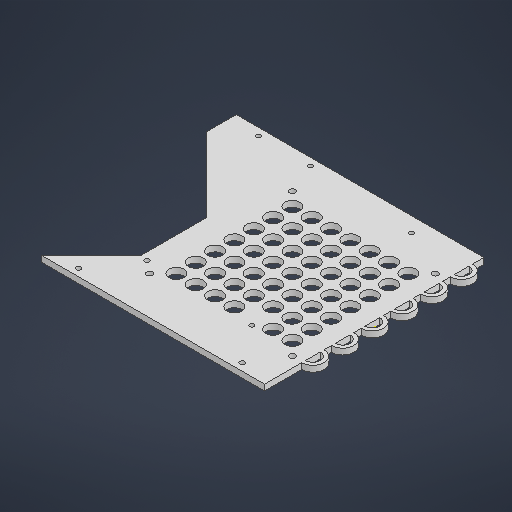
# Autodesk Inventor part: SidePlate_Ebox
Saved by Autodesk Inventor 2025.1 (Build 291241000, 241)
## iProperties
Created: 2025-03-19
Part Number: SidePlate_Ebox
Material: Generic
Document SubType Name: Modeling
Designer: m_kni
Density: 1 g/cm^3
Appearance: Default
Author: m_kni
Autodesk Inventor part; units mm, degrees
ref_plane "YZ Plane" through (0, 0, 0) normal (1, 0, 0) x (0, 1, 0)
ref_plane "XZ Plane" through (0, 0, 0) normal (0, 1, 0) x (-1, 0, 0)
ref_plane "XY Plane" through (0, 0, 0) normal (0, 0, 1) x (1, 0, 0)
sketch "Sketch1" plane through (0, 0, 0) normal (0, 1, 0) x (-1, 0, 0)
  line L0 (-83.0918, 73.8924) -> (-83.0918, -73.6076)
  line L1 (-83.0918, 73.8924) -> (-83.0918, -73.6076)
  line L2 (66.9082, 73.8924) -> (-83.0918, 73.8924)
  line L3 (-83.0918, 73.8924) -> (-83.0918, -73.6076)
  line L4 (-83.0918, -73.6076) -> (83.4082, -73.6076)
  line L5 (83.4082, -73.6076) -> (83.4082, -53.6076)
  line L6 (83.4082, -53.6076) -> (33.4082, -3.6076)
  line L7 (33.4082, -3.6076) -> (33.4082, 40.3924)
  line L8 (33.4082, 40.3924) -> (66.9082, 73.8924)
  point P0 (0, 0)
  point P1 (-8.0918, 73.8924)
  constraints: 18 end point, 1 vertical
extrude "Extrusion1" add sketch "Sketch1" along normal blind 4
sketch "Sketch2" plane through (0, 4, 0) normal (0, 1, 0) x (1, 0, 0)
  line L0 (83.0918, -73.8924) -> (83.0918, 73.6076) projected
  line L1 (-66.9082, -73.8924) -> (83.0918, -73.8924) projected
  line L2 (83.0918, -73.8924) -> (-66.9082, -73.8924)
  circle A0 centre (-46.9082, -68.8924) radius 1.6
  circle A1 centre (63.0918, -68.8924) radius 1.6
  point P0 (0, 0)
  dimension "d2" = 20
  dimension "d3" = 5
  dimension "d4" = 20
  dimension "d5" = 3.2
  dimension "d6" = 3.2
  constraints: 2 centre point, 2 coincident, 2 end point, 1 collinear
  measures "d2" horizontal distance of point (-46.908, -68.892) L1.start
  measures "d3" distance from line of L1 point (-46.908, -68.892)
  measures "d4" distance from line of point (63.092, -68.892) L0
  measures "d5" diameter of A0
  measures "d6" diameter of A1
extrude "Extrusion2" cut sketch "Sketch2" against normal blind 10
sketch "Sketch3" plane through (0, 4, 0) normal (0, 1, 0) x (1, 0, 0)
  line L0 (83.0918, 73.6076) -> (-83.4082, 73.6076) projected
  line L1 (-83.4082, 73.6076) -> (-83.4082, 53.6076) projected
  circle A0 centre (-63.4082, 68.6076) radius 1.5
  circle A1 centre (-28.4082, 68.6076) radius 1.5
  circle A2 centre (-28.4082, -41.3924) radius 1.5
  point P0 (0, 0)
  dimension "d9" = 5
  dimension "d10" = 20
  dimension "d11" = 3
  dimension "d12" = 35
  dimension "d13" = 110
  dimension "d14" = 3
  dimension "d15" = 3
  constraints: 3 centre point, 3 coincident
  measures "d9" distance from line of point (-63.408, 68.608) L0
  measures "d10" distance from line of L1 point (-63.408, 68.608)
  measures "d11" diameter of A0
  measures "d12" distance of point (-28.408, 68.608) A0.centre
  measures "d13" distance of point (-28.408, -41.392) point (-28.408, 68.608)
  measures "d14" diameter of A1
  measures "d15" diameter of A2
extrude "Extrusion3" cut sketch "Sketch3" against normal blind 10
sketch "Sketch4" plane through (0, 4, 0) normal (0, 1, 0) x (1, 0, 0)
  line L0 (83.0918, -73.8924) -> (83.0918, 73.6076) projected
  line L1 (-66.9082, -73.8924) -> (83.0918, -73.8924) projected
  circle A0 centre (44.5918, 63.6076) radius 1.5
  circle A1 centre (44.5918, -43.8924) radius 1.5
  point P0 (0, 0)
  dimension "d18" = 38.5
  dimension "d19" = 30
  dimension "d20" = 107.5
  dimension "d21" = 3
  dimension "d22" = 3
  constraints: 2 centre point, 2 coincident
  measures "d18" distance from line of L0 point (44.592, -43.892)
  measures "d19" distance from line of point (44.592, -43.892) L1
  measures "d20" distance of point (44.592, 63.608) point (44.592, -43.892)
  measures "d21" diameter of A0
  measures "d22" diameter of A1
extrude "Extrusion4" cut sketch "Sketch4" against normal blind 10
sketch "Sketch5" plane through (0, 4, 0) normal (0, 1, 0) x (1, 0, 0)
  line L0 (83.0918, -73.8924) -> (83.0918, 73.6076) projected
  line L1 (83.0918, -0.1424) -> (-26.9082, -0.1424)
  line L2 (-33.4082, 3.6076) -> (-33.4082, -40.3924) projected
  line L3 (83.0918, -55.1424) -> (-26.9082, -55.1424)
  line L4 (-26.9082, -55.1424) -> (-26.9082, 54.8576)
  line L5 (-26.9082, 54.8576) -> (83.0918, 54.8576)
  line L6 (83.0918, 54.8576) -> (83.0918, -55.1424)
  line L7 (83.0918, -55.1424) -> (-26.9082, 54.8576) construction
  line L8 (-26.9082, -55.1424) -> (83.0918, 54.8576) construction
  line L9 (76.0918, -48.1424) -> (-19.9082, -48.1424)
  line L10 (-19.9082, -48.1424) -> (-19.9082, 47.8576)
  line L11 (-19.9082, 47.8576) -> (76.0918, 47.8576)
  line L12 (76.0918, 47.8576) -> (76.0918, -48.1424)
  line L13 (76.0918, -48.1424) -> (-19.9082, 47.8576) construction
  line L14 (-19.9082, -48.1424) -> (76.0918, 47.8576) construction
  circle A0 centre (-19.9082, 47.8576) radius 2
  circle A1 centre (76.0918, 47.8576) radius 2
  circle A2 centre (-19.9082, -48.1424) radius 2
  circle A3 centre (76.0918, -48.1424) radius 2
  circle A4 centre (-11.0143, 38.9637) radius 5
  circle A5 centre (-11.0143, 25.9637) radius 5
  circle A6 centre (-11.0143, 12.9637) radius 5
  circle A7 centre (-11.0143, -0.0363) radius 5
  circle A8 centre (-11.0143, -13.0363) radius 5
  circle A9 centre (-11.0143, -26.0363) radius 5
  circle A10 centre (-11.0143, -39.0363) radius 5
  circle A11 centre (1.9857, 38.9637) radius 5
  circle A12 centre (1.9857, 25.9637) radius 5
  circle A13 centre (1.9857, 12.9637) radius 5
  circle A14 centre (1.9857, -0.0363) radius 5
  circle A15 centre (1.9857, -13.0363) radius 5
  circle A16 centre (1.9857, -26.0363) radius 5
  circle A17 centre (1.9857, -39.0363) radius 5
  circle A18 centre (14.9857, 38.9637) radius 5
  circle A19 centre (14.9857, 25.9637) radius 5
  circle A20 centre (14.9857, 12.9637) radius 5
  circle A21 centre (14.9857, -0.0363) radius 5
  circle A22 centre (14.9857, -13.0363) radius 5
  circle A23 centre (14.9857, -26.0363) radius 5
  circle A24 centre (14.9857, -39.0363) radius 5
  circle A25 centre (27.9857, 38.9637) radius 5
  circle A26 centre (27.9857, 25.9637) radius 5
  circle A27 centre (27.9857, 12.9637) radius 5
  circle A28 centre (27.9857, -0.0363) radius 5
  circle A29 centre (27.9857, -13.0363) radius 5
  circle A30 centre (27.9857, -26.0363) radius 5
  circle A31 centre (27.9857, -39.0363) radius 5
  circle A32 centre (40.9857, 38.9637) radius 5
  circle A33 centre (40.9857, 25.9637) radius 5
  circle A34 centre (40.9857, 12.9637) radius 5
  circle A35 centre (40.9857, -0.0363) radius 5
  circle A36 centre (40.9857, -13.0363) radius 5
  circle A37 centre (40.9857, -26.0363) radius 5
  circle A38 centre (40.9857, -39.0363) radius 5
  circle A39 centre (53.9857, 38.9637) radius 5
  circle A40 centre (53.9857, 25.9637) radius 5
  circle A41 centre (53.9857, 12.9637) radius 5
  circle A42 centre (53.9857, -0.0363) radius 5
  circle A43 centre (53.9857, -13.0363) radius 5
  circle A44 centre (53.9857, -26.0363) radius 5
  circle A45 centre (53.9857, -39.0363) radius 5
  circle A46 centre (66.9857, 38.9637) radius 5
  circle A47 centre (66.9857, 25.9637) radius 5
  circle A48 centre (66.9857, 12.9637) radius 5
  circle A49 centre (66.9857, -0.0363) radius 5
  circle A50 centre (66.9857, -13.0363) radius 5
  circle A51 centre (66.9857, -26.0363) radius 5
  circle A52 centre (66.9857, -39.0363) radius 5
  point P0 (0, 0)
  point P1 (28.0918, -0.1424)
  dimension "d25" = 110
  dimension "d26" = 110
  dimension "d27" = 96
  dimension "d28" = 96
  dimension "d29" = 4
  dimension "d30" = 4
  dimension "d31" = 4
  dimension "d32" = 4
  dimension "d33" = 10
  dimension "d36" = 13
  dimension "d39" = 13
  constraints: 53 centre point, 26 end point, 6 midpoint, 4 coincident, 4 parallel, 3 horizontal, 3 perpendicular, 1 point on line, 1 vertical, 96 other
  measures "d25" distance of L1.start L1.end
  measures "d26" distance of L3.end L4.end
  measures "d27" distance of L10.end L11.end
  measures "d28" distance of L9.end L10.end
  measures "d29" diameter of A0
  measures "d30" diameter of A1
  measures "d31" diameter of A2
  measures "d32" diameter of A3
  measures "d33" diameter of A4
  measures "d36" distance of A4.centre A5.centre
  measures "d39" distance of A4.centre A11.centre
extrude "Extrusion5" cut sketch "Sketch5" against normal blind 10 contours A49 L1 | L1 A49 | A1 L11 L12 | L12 L11 A1 | A3 L9 L12 | L12 L9 A3 | A7 L1 | L1 A7 | A2 L9 L10 | L10 L9 A2 | A0 L11 L10 | L10 L11 A0 | A42 L1 | L1 A42 | A14 L1 | L1 A14 | A35 L1 | L1 A35 | A21 L1 | L1 A21 | A28 L1 | L1 A28 | A4 | A5 | A6 | A8 | A9 | A10 | A11 | A12 | A13 | A15 | A16 | A17 | A18 | A19 | A20 | A22 | A23 | A24 | A25 | A26 | A27 | A29 | A30 | A31 | A32 | A33 | A34 | A36 | A37 | A39 | A40 | A41 | A43 | A44 | A45 | A46 | A47 | A48 | A50 | A51 | A52
sketch "Sketch6" plane through (83.0918, 0, 73.8924) normal (1, 0, 0) x (0, 0, -1)
  point P0 (73.8924, 0)
sketch "Sketch7" plane through (0, 4, 0) normal (0, 1, 0) x (1, 0, 0)
  line L0 (83.0918, -73.8924) -> (83.0918, 73.6076) projected
  line L1 (83.0918, 73.6076) -> (-83.4082, 73.6076) projected
  circle A0 centre (83.0918, 58.6076) radius 5
  circle A1 centre (83.0918, 58.6076) radius 7.5
  circle A2 centre (83.0918, 38.6076) radius 5
  circle A3 centre (83.0918, 38.6076) radius 7.5
  circle A4 centre (83.0918, 18.6076) radius 5
  circle A5 centre (83.0918, 18.6076) radius 7.5
  circle A6 centre (83.0918, -1.3924) radius 5
  circle A7 centre (83.0918, -1.3924) radius 7.5
  circle A8 centre (83.0918, -21.3924) radius 5
  circle A9 centre (83.0918, -21.3924) radius 7.5
  circle A10 centre (83.0918, -41.3924) radius 5
  circle A11 centre (83.0918, -41.3924) radius 7.5
  line L2 (83.0918, 66.1076) -> (83.0918, -48.8924)
  point P0 (0, 0)
  point P1 (83.0918, -33.8924)
  point P2 (83.0918, -36.3924)
  point P3 (83.0918, -46.3924)
  point P4 (83.0918, -13.8924)
  point P5 (83.0918, -16.3924)
  point P6 (83.0918, -26.3924)
  point P7 (83.0918, -28.8924)
  point P8 (83.0918, 6.1076)
  point P9 (83.0918, 3.6076)
  point P10 (83.0918, -6.3924)
  point P11 (83.0918, -8.8924)
  point P12 (83.0918, 26.1076)
  point P13 (83.0918, 23.6076)
  point P14 (83.0918, 13.6076)
  point P15 (83.0918, 11.1076)
  point P16 (83.0918, 46.1076)
  point P17 (83.0918, 43.6076)
  point P18 (83.0918, 33.6076)
  point P19 (83.0918, 31.1076)
  point P20 (83.0918, 63.6076)
  point P21 (83.0918, 53.6076)
  point P22 (83.0918, 51.1076)
  dimension "d46" = 15
  dimension "d44" = 15
  dimension "d45" = 10
  dimension "d49" = 20
  constraints: 10 centre point, 10 vertical alignment, 8 equal radius, 7 coincident, 2 end point, 12 other
  measures "d44" distance from line of point (83.092, 58.608) L1
  measures "d45" diameter of A0
  measures "d49" distance of A0.centre A2.centre
extrude "Extrusion6" add sketch "Sketch7" against normal up to surface (4 mm away) contours L0 A10 A11 | L0 A8 A9 | L0 A6 A7 | L0 A4 A5 | L0 A2 A3 | L0 A0 A1 picked at (89.654, -40.4652) picked at (89.654, -22.3196) picked at (89.654, -2.3196) picked at (89.654, 17.6804) picked at (89.654, 37.6804) picked at (89.654, 57.6804)
body "Solid1"
